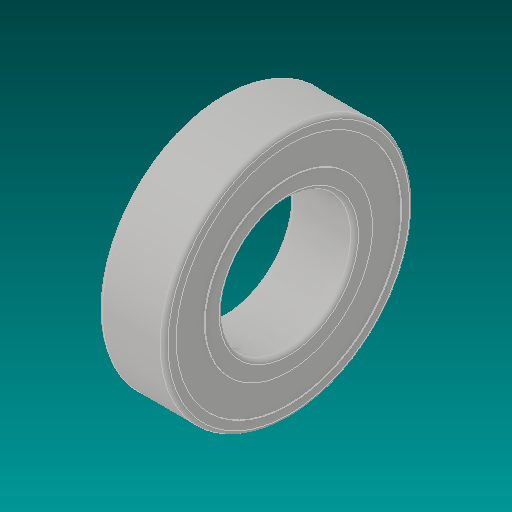
# Autodesk Inventor part: bearing_6800
Saved by Autodesk Inventor 2020 (Build 240168000, 168)
## iProperties
Created: 2022-11-02
Part Number: bearing_6800
Material: Generic
Catalog Web Link: www.cadenas.de
Description: 6000_bearing-Deep Groove Ball Bearings
Vendor: MISUMI
Document SubType Name: Modeling
Designer: psAdmin
Manufacturer: MISUMI
Mass: 1.00952 g
Surface Area: 8.52846 cm^2
Volume: 1.00952 cm^3
Density: 1 g/cm^3
Appearance: PSOLRGB-175-175-175
Category: PARTsolutions
Company: MISUMI
PSOL_IDENT_0: {$CADENAS_DATA/23d-libs/misumi/metric/accessories/bearing_6000.prj},170 {VTYP=3D},{NB=bearing_6800},
PSOL_IDENT_1: {LINA=bearing_6800},{NN=6000_bearing},{DATE=30.06.2021 13:30:08},{GEOMDATE=24.10.2013 00:00:00},{VER
PSOL_IDENT_2: SION=},{LINEID=20},{WBVAR=},{WBNUMERIC=}  {NB=bearing_6800},{LINA=bearing_6800},{KT=DUMMY},{PN=beari
PSOL_IDENT_3: ng_6800},{BN=6800},{DD=10},{D=19},{B=5},{RR=0.3},{DSMIN=12.0},{DS1=12.50},{DSMAX=12.50},{DDHH=17.0},
PSOL_IDENT_4: {R=0.3},{R1=1.000},{R2=1.000},{MASS=5},{MASS11=5},{AA=4.8850},{BB=0.9250},{CC=1.3700},{DD1=1.000}
NB: bearing_6800
NN: 6000_bearing
NT: Deep Groove Ball Bearings
NBSYN: $PN.
LINA: bearing_6800
CATALOG: Misumi
PN: bearing_6800
BN: 6800
DD: 10
D: 19
B: 5
RR: 0.3
DSMIN: 12
DDHH: 17
R: 0.3
MASS11: 5
SUPPLIER: MISUMI
ARTICLENO: bearing_6800
BOMINFO: bearing_6800
CREATOR: CADENAS GmbH
d1: 0.000 mm
Title: bearing_6800
Author: Cadenas PARTsolutions
Comments: Deep Groove Ball Bearings
Autodesk Inventor part; units mm, degrees
ref_plane "YZ Plane" through (0, 0, 0) normal (1, 0, 0) x (0, 1, 0)
ref_plane "XZ Plane" through (0, 0, 0) normal (0, 1, 0) x (-1, 0, 0)
ref_plane "XY Plane" through (0, 0, 0) normal (0, 0, 1) x (1, 0, 0)
sketch "Sketch_1" plane through (0, 0, 0) normal (0, 0, 1) x (1, 0, 0)
  line L0 (5, 0) -> (0, 0)
  arc A0 (0, 5.3) -> (0.3, 5) centre (0.3, 5.3) ccw
  line L1 (0.3, 5) -> (4.7, 5)
  arc A1 (4.7, 5) -> (5, 5.3) centre (4.7, 5.3) ccw
  line L2 (5, 5.3) -> (5, 6.37)
  line L3 (5, 6.37) -> (4.9425, 6.37)
  line L4 (4.9425, 6.37) -> (4.9425, 8.575)
  line L5 (4.9425, 8.575) -> (5, 8.575)
  line L6 (5, 8.575) -> (5, 9.2)
  arc A2 (5, 9.2) -> (4.7, 9.5) centre (4.7, 9.2) ccw
  line L7 (4.7, 9.5) -> (0.3, 9.5)
  arc A3 (0.3, 9.5) -> (0, 9.2) centre (0.3, 9.2) ccw
  line L8 (0, 9.2) -> (0, 8.575)
  line L9 (0, 8.575) -> (0.0575, 8.575)
  line L10 (0.0575, 8.575) -> (0.0575, 6.37)
  line L11 (0.0575, 6.37) -> (0, 6.37)
  line L12 (0, 6.37) -> (0, 5.3)
  constraints: 26 end point, 8 point on circle, 4 centre point
revolve "Revolution1" add sketch "Sketch_1" angle 360 about axis through (5, 0, 0) along (1, 0, 0)
ref_plane "center_point_XY" through (2.5, 0, 0) normal (1, 0, 0) x (0, 0, -1)
ref_plane "center_point_YZ" through (2.5, 0, 0) normal (0, 0, -1) x (0, 1, 0)
ref_plane "center_point_ZX" through (2.5, 0, 0) normal (0, 1, 0) x (1, 0, 0)
ref_plane "to_housing_XY" through (0, 0, 0) normal (1, 0, 0) x (0, 0, -1)
ref_plane "to_housing_YZ" through (0, 0, 0) normal (0, 0, -1) x (0, 1, 0)
ref_plane "to_housing_ZX" through (0, 0, 0) normal (0, 1, 0) x (1, 0, 0)
ref_plane "to_ring_XY" through (4.885, 0, 0) normal (1, 0, 0) x (0, 0, -1)
ref_plane "to_ring_YZ" through (4.885, 0, 0) normal (0, 0, -1) x (0, 1, 0)
ref_plane "to_ring_ZX" through (4.885, 0, 0) normal (0, 1, 0) x (1, 0, 0)
body "Solid1"
